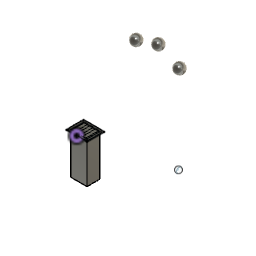
Installation v1 v6 (Autodesk Fusion 360 design; units mm, degrees)
Autodesk Fusion 360 part; units mm, degrees
ref_plane "WorkPlane1" through (0, 0, 1200) normal (0, 0, 1) x (1, 0, 0)
sketch "Sketch1" plane through (0, 0, 1200) normal (0, 0, 1) x (1, 0, 0) in component "Table"
  line L0 (-300, 500) -> (300, 500)
  line L1 (300, 500) -> (300, 0)
  line L2 (300, 0) -> (-300, 0)
  line L3 (-300, 0) -> (-300, 500)
  line L4 (-240, 440) -> (240, 440)
  line L5 (240, 440) -> (240, 60)
  line L6 (240, 60) -> (-240, 60)
  line L7 (-240, 60) -> (-240, 440)
  dimension "d1" = 600
  dimension "d2" = 500
  dimension "d27" = 60
  constraint horizontal L0
  constraint vertical L1
  constraint horizontal L2
  constraint vertical L3
  constraint midpoint origin L2
  measures "d1" distance of L0.start L0.end
  measures "d2" distance of L0.start L2.end
extrude "Extrude1" add sketch "Sketch1" along normal blind 16 contours L0 L1 L2 L3 | L4 L5 L6 L7 makes body 1 in component "Table"
fillet "Fillet1" radius 100 4 edges at (-300, 0, 1208) (300, 0, 1208) (300, 500, 1208) (-300, 500, 1208) on bodies 1 in component "Table"
sketch "Sketch1 (2)" plane through (0, 0, 1216) normal (0, 0, 1) x (-1, 0, 0) in component "MetalPlate"
  arc A0 (200, -500) -> (300, -400) centre (200, -400) ccw
  line L0 (300, -400) -> (300, -100)
  arc A1 (300, -100) -> (200, 0) centre (200, -100) ccw
  line L1 (200, 0) -> (-200, 0)
  arc A2 (-200, 0) -> (-300, -100) centre (-200, -100) ccw
  line L2 (-300, -100) -> (-300, -400)
  arc A3 (-300, -400) -> (-200, -500) centre (-200, -400) ccw
  line L3 (-200, -500) -> (200, -500)
  line L4 (45.491, -450) -> (-44.509, -450)
  line L5 (-44.509, -450) -> (-44.509, -50)
  line L6 (-44.509, -50) -> (45.491, -50)
  line L7 (45.491, -50) -> (45.491, -450)
  point P0 (0.491, -450)
  dimension "d16" = 90
  dimension "d17" = 400
  dimension "d18" = 50
  constraint horizontal L4
  constraint vertical L5
  constraint horizontal L6
  constraint vertical L7
  constraint midpoint L4 P0
  measures "d16" distance of L4.start L4.end
  measures "d17" distance of L4.start L6.end
  measures "d18" distance of L3 L4
extrude "Extrude1'" add sketch "Sketch1 (2)" along normal blind 1 separate body contours L4 L5 L6 L7 makes body 2 in component "MetalPlate"
pattern_linear "00000000-0000-0000-0000-000000000000" [suppressed]
fillet "Fillet1'" radius 30 4 edges at (44.509, 50, 1216.5) (-45.491, 50, 1216.5) (44.509, 450, 1216.5) (-45.491, 450, 1216.5) on bodies 2 in component "MetalPlate"
sketch "Sketch1 (3)" plane through (0, 0, 0) normal (0, 0, 1) x (1, 0, 0) in component "Table stand"
extrude "Extrude4" add sketch "Sketch1" against normal blind 1200 contours L4 L5 L6 L7 bodies 1 in component "Table"
shell "Shell1" thickness 10 removed faces 1 at (-80, 313.3333, 0) on bodies 1 in component "Table"
sphere "SpherePrimitive1" add diameter 300 placed x (-1, 0, 0) y (0, -1, 0) z (0, 0, 1) at (184.1388, 600.8855, 1216) separate body makes body 3 in component "Floating 1"
pattern_linear "00000000-0000-0000-0000-000000000000'" [suppressed]
sketch "Sketch1 (4)" plane through (0, 0, 0) normal (1, 0, 0) x (0, 1, 0) in component "rope wheel"
  circle A0 centre (2975.7259, -1150.238) radius 60
  circle A1 centre (2975.7259, -1150.238) radius 20
  dimension "d41" = 120
  dimension "d42" = -40
  measures "d41" diameter of A0
extrude "Extrude1''" add sketch "Sketch1 (4)" along normal blind 5 separate body contours A0 | A1 makes body 4 in component "rope wheel"
extrude "Extrude3" add sketch "Sketch1 (4)" against normal blind 20 contours A1 bodies 4 in component "rope wheel"
component "Table" placed x (1, 0, 0) y (0, 1, 0) z (0, 0, 1) at (0, 0, 0)
component "MetalPlate" placed x (1, 0, 0) y (0, 1, 0) z (0, 0, 1) at (0, 0, 0)
component "MetalPlate" placed x (1, 0, 0) y (0, 1, 0) z (0, 0, 1) at (-160, 0, 0)
component "MetalPlate" placed x (1, 0, 0) y (0, 1, 0) z (0, 0, 1) at (160, 0, 0)
component "Table stand" placed x (1, 0, 0) y (0, 1, 0) z (0, 0, 1) at (0, 0, 0)
component "Floating 1" placed x (1, 0, 0) y (0, 1, 0) z (0, 0, 1) at (-189.4101, 1791.4129, 1105.6874)
component "Floating 1" placed x (1, 0, 0) y (0, 1, 0) z (0, 0, 1) at (429.9657, 1791.4129, 807.2999)
component "Floating 1" placed x (1, 0, 0) y (0, 1, 0) z (0, 0, 1) at (-835.9121, 1791.4129, 892.5535)
component "rope wheel" placed x (1, 0, 0) y (0, 1, 0) z (0, 0, 1) at (0, 0, 0)
